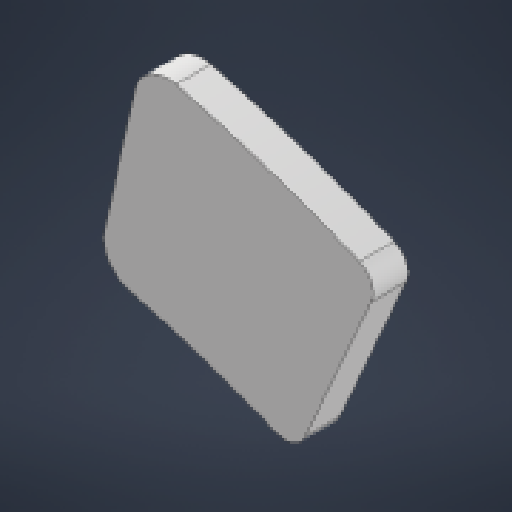
# Autodesk Inventor part: 斜板固定件
Saved by Autodesk Inventor 2025 (Build 290162000, 162)
## iProperties
Created: 2025-01-08
Part Number: 斜板固定件
Material: 常规
Document SubType Name: Modeling
Designer: HZD
Density: 1 g/cm^3
Appearance: 默认
Author: HZD
Autodesk Inventor part; units mm, degrees
ref_plane "YZ Plane" through (0, 0, 0) normal (1, 0, 0) x (0, 1, 0)
ref_plane "XZ Plane" through (0, 0, 0) normal (0, 1, 0) x (-1, 0, 0)
ref_plane "XY Plane" through (0, 0, 0) normal (0, 0, 1) x (1, 0, 0)
sketch "草图2" plane through (0, 0, 0) normal (0, 0, 1) x (1, 0, 0)
  arc A0 (11.812, -10.0858) -> (14.4114, -9.0466) centre (12.5814, -8.2397) ccw projected
  arc A1 (11.812, -10.0858) -> (-0.838, -5.8193) centre (-25.1186, -98.698) ccw projected
  arc A2 (-3.01, -2.276) -> (-0.838, -5.8193) centre (-0.0792, -2.9169) ccw projected
  line L0 (-0.4446, 9.4555) -> (-3.01, -2.276) projected
  arc A3 (3.2323, 11.7204) -> (-0.4446, 9.4555) centre (2.4862, 8.8147) ccw projected
  arc A4 (19.0048, 6.4168) -> (3.2323, 11.7204) centre (-25.1186, -98.698) ccw projected
  arc A5 (20.0607, 3.7658) -> (19.0048, 6.4168) centre (18.2307, 4.5727) ccw projected
  line L1 (14.4114, -9.0466) -> (20.0607, 3.7658) projected
  arc A6 (19.9692, 3.8061) -> (18.9661, 6.3246) centre (18.2307, 4.5727) ccw
  arc A7 (18.9661, 6.3246) -> (3.2074, 11.6235) centre (-25.1186, -98.698) ccw
  arc A8 (3.2074, 11.6235) -> (-0.3469, 9.4342) centre (2.4862, 8.8147) ccw
  line L2 (-0.3469, 9.4342) -> (-2.9123, -2.2974)
  arc A9 (-2.9123, -2.2974) -> (-0.8127, -5.7226) centre (-0.0792, -2.9169) ccw
  arc A10 (11.8505, -9.9935) -> (-0.8127, -5.7226) centre (-25.1186, -98.698) ccw
  arc A11 (11.8505, -9.9935) -> (14.3199, -9.0062) centre (12.5814, -8.2397) ccw
  line L3 (14.3199, -9.0062) -> (19.9692, 3.8061)
  dimension "d2" = 0.1
  constraints: 12 point on circle, 6 centre point, 4 end point, 7 other
  measures "d2" distance between parallel lines of L1 L3
extrude "拉伸1" add sketch "草图2" along normal blind 3 contours L3 A11 A10 A9 L2 A8 A7 A6
